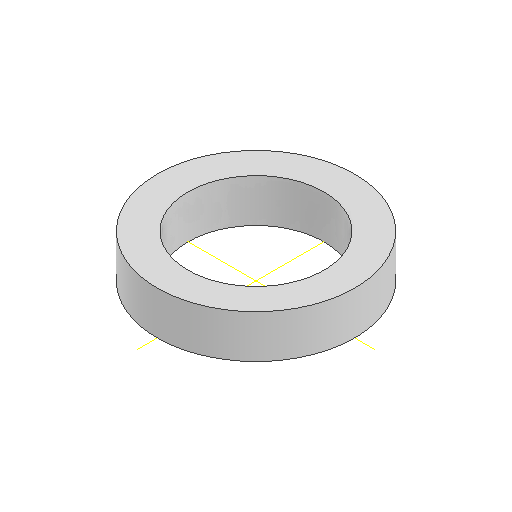
# Autodesk Inventor part: 베어링
Saved by Autodesk Inventor 2027 (Build 310192000, 192)
## iProperties
Created: 2026-09-17
Part Number: 베어링
Material: 일반
Document SubType Name: Modeling
Designer: User
Density: 1 g/cm^3
Appearance: 기본값
Author: User
Autodesk Inventor part; units mm, degrees
ref_plane "YZ 평면_우측면도" through (0, 0, 0) normal (1, 0, 0) x (0, 1, 0)
ref_plane "XZ 평면_평면도" through (0, 0, 0) normal (0, 1, 0) x (-1, 0, 0)
ref_plane "XY 평면_정면도" through (0, 0, 0) normal (0, 0, 1) x (1, 0, 0)
sketch "스케치1" plane through (0, 0, 0) normal (0, 1, 0) x (-1, 0, 0)
  circle A0 centre (0, 0) radius 16
  circle A1 centre (0, 0) radius 11
  dimension "d0" = 32
  dimension "d1" = 22
  constraints: 2 centre point, 2 coincident
  measures "d0" diameter of A0
  measures "d1" diameter of A1
extrude "돌출1" add sketch "스케치1" along normal blind 7
